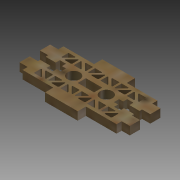
# Autodesk Inventor part: ESCcableHolder
Saved by Autodesk Inventor 2012 (Build 160160000, 160)
## iProperties
Created: 2014-07-18
Part Number: ESCcableHolder
Material: Default
Document SubType Name: Modeling
Designer: Anon
Density: 1 g/cm^3
GlobalPropertyList: <PropertyList/>
Author: Anon
Autodesk Inventor part; units mm, degrees
ref_plane "YZ Plane" through (0, 0, 0) normal (1, 0, 0) x (0, 1, 0)
ref_plane "XZ Plane" through (0, 0, 0) normal (0, 1, 0) x (-1, 0, 0)
sketch "Sketch1" plane through (0, 0, 0) normal (0, 0, 1) x (1, 0, 0)
  line L0 (-23, 10) -> (-8, 10)
  line L1 (-8, 10) -> (-8, 14)
  line L2 (-23, 10) -> (-23, 7.5)
  line L3 (-23, 7.5) -> (-27, 7.5)
  line L4 (-27, 7.5) -> (-27, 2.5)
  line L5 (-27, 2.5) -> (-23, 2.5)
  line L6 (-23, 2.5) -> (-23, 0)
  line L7 (-23, 0) -> (0, 0)
  line L8 (0, 0) -> (0, 14)
  line L9 (0, 14) -> (-8, 14)
  line L10 (-23, -10) -> (-8, -10)
  line L11 (-8, -10) -> (-8, -14)
  line L12 (-23, -10) -> (-23, -7.5)
  line L13 (-23, -7.5) -> (-27, -7.5)
  line L14 (-27, -7.5) -> (-27, -2.5)
  line L15 (-27, -2.5) -> (-23, -2.5)
  line L16 (-23, -2.5) -> (-23, 0)
  line L17 (0, 0) -> (0, -14)
  line L18 (0, -14) -> (-8, -14)
  line L19 (23, 10) -> (8, 10)
  line L20 (8, 10) -> (8, 14)
  line L21 (23, 10) -> (23, 7.5)
  line L22 (23, 7.5) -> (27, 7.5)
  line L23 (27, 7.5) -> (27, 2.5)
  line L24 (27, 2.5) -> (23, 2.5)
  line L25 (23, 2.5) -> (23, 0)
  line L26 (23, 0) -> (0, 0)
  line L27 (0, 14) -> (8, 14)
  line L28 (23, -10) -> (8, -10)
  line L29 (8, -10) -> (8, -14)
  line L30 (23, -10) -> (23, -7.5)
  line L31 (23, -7.5) -> (27, -7.5)
  line L32 (27, -7.5) -> (27, -2.5)
  line L33 (27, -2.5) -> (23, -2.5)
  line L34 (23, -2.5) -> (23, 0)
  line L35 (0, -14) -> (8, -14)
  dimension "d0" = 15
  dimension "d1" = 4
  dimension "d118" = 2.5
  dimension "d119" = 4
  dimension "d120" = 5
  dimension "d121" = 4
  constraints: 72 end point, 23 symmetric about line, 5 parallel, 2 perpendicular, 1 collinear, 1 horizontal
  measures "d0" distance of L0.start L0.end
  measures "d1" distance of L0.end L1.end
  measures "d118" distance of L0.start L2.end
  measures "d119" distance of L2.end L3.end
  measures "d120" distance of L3.end L4.end
  measures "d121" distance of L4.end L5.end
extrude "Contour" add sketch "Sketch1" along normal blind 4
sketch "Sketch11" plane through (0, 0, 4) normal (0, 0, 1) x (1, 0, 0)
  line L0 (-23, -2.5) -> (-23, 2.5) projected
  line L1 (-8, -14) -> (-8, -10) projected
  line L2 (-23, 1.25) -> (-18, 1.25)
  line L3 (-18, 1.25) -> (-18, 3.25)
  line L4 (-18, 3.25) -> (-15, 3.25)
  line L5 (-15, 3.25) -> (-15, 1.25)
  line L6 (-15, 1.25) -> (-13, 1.25)
  line L7 (-13, 1.25) -> (-13, -1.25)
  line L8 (-13, -1.25) -> (-15, -1.25)
  line L9 (-15, -1.25) -> (-15, -3.25)
  line L10 (-15, -3.25) -> (-18, -3.25)
  line L11 (-18, -3.25) -> (-18, -1.401)
  line L12 (-18, -1.401) -> (-23, -1.401)
  line L13 (-23, 1.25) -> (-23, -1.401)
  point P0 (0, 0)
  dimension "d122" = 5
  dimension "d123" = 2
  dimension "d124" = 3
  dimension "d125" = 2
  dimension "d126" = 2
  dimension "d127" = 2.5
  dimension "d128" = 2
  dimension "d129" = 1.25
  dimension "d130" = 2
  constraints: 24 end point, 6 parallel, 3 collinear, 3 perpendicular, 2 point on line
  measures "d122" distance of L2.start L2.end
  measures "d123" distance of L2.end L3.end
  measures "d124" distance of L3.end L4.end
  measures "d125" distance of L4.end L5.end
  measures "d126" distance of L5.end L6.end
  measures "d127" distance of L6.end L7.end
  measures "d128" distance of L8.end L9.end
  measures "d129" distance from line of point (0, 0) L2
  measures "d130" distance of L7.end L8.end
extrude "ScrewLock" cut sketch "Sketch11" against normal blind 4
mirror "ScrewLockDoubler" about plane through (0, 0, 0) normal (1, 0, 0) of "ScrewLock"
sketch "Sketch12" plane through (0, 0, 4) normal (0, 0, 1) x (1, 0, 0)
  line L0 (-8, 14) -> (8, 14) projected
  line L1 (8, -14) -> (-8, -14) projected
  line L2 (0, 14) -> (0, -14) construction
  point P0 (0, 0)
  point P1 (-8, 0)
  point P2 (8, 0)
  dimension "d133" = 8
  constraints: 2 end point, 2 midpoint, 1 symmetric about line
  measures "d133" distance of point (0, 0) point (-8, 0)
hole "CableHoles" at (-8, 0, 4) at (8, 0, 4) direction (0, 0, -1) diameter 6 end through all
sketch "Sketch15" plane through (0, 0, 4) normal (0, 0, 1) x (1, 0, 0)
  line L0 (18, 3.25) -> (18, 1.25) projected
  line L1 (-19, 8.5) -> (-19, 4.5)
  line L2 (-15, 8.5) -> (-19, 8.5)
  line L3 (-19, 4.5) -> (-15, 8.5)
  line L4 (-13.5, 8.5) -> (-13.5, 4.5)
  line L5 (-13.5, 4.5) -> (-17.5, 4.5)
  line L6 (-17.5, 4.5) -> (-13.5, 8.5)
  line L7 (-23, 10) -> (-8, 10) projected
  line L8 (-23, 7.5) -> (-23, 10) projected
  point P0 (0, 0)
  dimension "d147" = 4
  dimension "d149" = 4
  dimension "d150" = 1.5
  dimension "d158" = 4
  dimension "d159" = 4
  dimension "d160" = 1.5
  constraints: 12 end point, 3 perpendicular, 2 parallel
  measures "d147" distance of L1.start L1.end
  measures "d149" distance of L4.end L5.end
  measures "d150" distance of L4.start L2.start
  measures "d158" distance of L4.start L4.end
  measures "d159" distance between parallel lines of L8 L1
  measures "d160" distance between parallel lines of L7 L2
extrude "FillPattern" cut sketch "Sketch15" against normal blind 4
fillet "FillPatternFillet" radius 0.3 6 edges at (-19, 8.5, 2) (-15, 8.5, 2) (-13.5, 8.5, 2) (-19, 4.5, 2) (-17.5, 4.5, 2) (-13.5, 4.5, 2)
ref_plane "FillPatternMirror" through (-13, 4.8, 4) normal (-1, 0, 0) x (0, 0, 1)
mirror "FillPatternSquare" about plane through (-13, 4.8, 4) normal (-1, 0, 0) of "FillPattern", "FillPatternFillet"
pattern_linear "FillPatternSpread" count 3 spacing 13 along (1, 0, 0) of "FillPattern", "FillPatternFillet", "FillPatternSquare"
mirror "FillPatternDoubler" about plane through (0, 0, 0) normal (0, 1, 0) of "FillPattern", "FillPatternFillet", "FillPatternSquare", "FillPatternSpread"
sketch "Sketch16" plane through (0, 0, 4) normal (0, 0, 1) x (1, 0, 0)
  line L0 (-4, 2) -> (4, 2)
  line L1 (4, 2) -> (4, -2)
  line L2 (4, -2) -> (-4, -2)
  line L3 (-4, -2) -> (-4, 2)
  point P0 (0, 0)
  dimension "d161" = 4
  dimension "d162" = 8
  dimension "d163" = 4
  dimension "d164" = 2
  constraints: 8 end point, 2 parallel, 1 horizontal, 1 perpendicular
  measures "d161" distance between parallel lines of L0 L2
  measures "d162" distance between parallel lines of L1 L3
  measures "d163" distance from line of point (0, 0) L1
  measures "d164" distance from line of point (0, 0) L0
extrude "ServoCableHole" cut sketch "Sketch16" against normal blind 4
body "Solid1"
